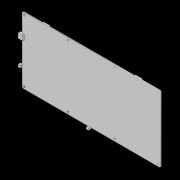
# Autodesk Inventor part: seaboard-block-circuit-board
Saved by Autodesk Inventor 2020 (Build 240168000, 168)
## iProperties
Created: 2019-06-07
Part Number: seaboard-block-circuit-board
Material: Generic
Document SubType Name: Modeling
Designer: valer
Density: 1 g/cm^3
Appearance: Default
Author: valer
Autodesk Inventor part; units mm, degrees
ref_plane "YZ Plane" through (0, 0, 0) normal (1, 0, 0) x (0, 1, 0)
ref_plane "XZ Plane" through (0, 0, 0) normal (0, 1, 0) x (-1, 0, 0)
ref_plane "XY Plane" through (0, 0, 0) normal (0, 0, 1) x (1, 0, 0)
sketch "CircuitBoard" plane through (0, 0, 0) normal (0, 0, 1) x (1, 0, 0)
  line L0 (-271.4625, 131.7625) -> (-267.0175, 131.7625) construction
  line L1 (0, 129.3813) -> (0, 5.9531)
  line L2 (0, 0) -> (-267.0175, 0) construction
  line L3 (-271.4625, 0) -> (-271.4625, 131.7625) construction
  line L4 (-271.4625, 95.25) -> (-267.0175, 95.25)
  line L5 (-267.0175, 95.25) -> (-267.0175, 86.1219) construction
  line L6 (-267.0175, 86.1219) -> (-271.4625, 86.1219)
  line L7 (-271.4625, 86.1219) -> (-271.4625, 95.25)
  line L8 (-271.4625, 95.25) -> (-262.3344, 95.25)
  line L9 (-262.3344, 95.25) -> (-262.3344, 86.1219)
  line L10 (-262.3344, 86.1219) -> (-271.4625, 86.1219)
  line L11 (-271.4625, 86.1219) -> (-271.4625, 95.25)
  line L12 (-267.0175, 95.25) -> (-267.0175, 129.3813)
  line L13 (-264.6363, 131.7625) -> (-2.3812, 131.7625)
  line L14 (-267.0175, 86.1219) -> (-267.0175, 5.9531)
  line L15 (-267.0175, 0) -> (-271.4625, 0) construction
  line L16 (-135.255, 0) -> (-140.0175, 0)
  line L17 (-140.0175, 0) -> (-140.0175, 3.5719)
  line L18 (-140.0175, 3.5719) -> (-135.255, 3.5719)
  line L19 (-135.255, 3.5719) -> (-135.255, 0)
  line L20 (-140.0175, 0) -> (-135.255, 0)
  line L21 (-135.255, 0) -> (-135.255, -1.5875)
  line L22 (-135.255, -1.5875) -> (-140.0175, -1.5875)
  line L23 (-140.0175, -1.5875) -> (-140.0175, 0)
  line L24 (-271.4625, 42.8625) -> (-267.0175, 42.8625)
  line L25 (-267.0175, 42.8625) -> (-267.0175, 38.1)
  line L26 (-267.0175, 38.1) -> (-271.4625, 38.1)
  line L27 (-271.4625, 38.1) -> (-271.4625, 42.8625)
  circle A0 centre (-262.8456, 127.5906) radius 1.7859
  arc A1 (-264.6363, 131.7625) -> (-267.0175, 129.3813) centre (-264.6362, 129.3813) ccw
  arc A2 (0, 129.3813) -> (-2.3812, 131.7625) centre (-2.3812, 129.3813) ccw
  circle A3 centre (-178.7081, 127.5906) radius 1.7859
  line L28 (-262.8456, 127.5906) -> (-178.7081, 127.5906) construction
  line L29 (-271.4625, 42.8625) -> (-273.05, 42.8625)
  line L30 (-273.05, 42.8625) -> (-273.05, 38.1)
  line L31 (-273.05, 38.1) -> (-271.4625, 38.1)
  line L32 (-271.4625, 38.1) -> (-271.4625, 42.8625)
  line L33 (-140.0175, 3.5719) -> (-264.6363, 3.5719)
  line L34 (-135.255, 3.5719) -> (-2.3813, 3.5719)
  line L35 (0, 3.5719) -> (0, 0) construction
  arc A4 (-267.0175, 5.9531) -> (-264.6363, 3.5719) centre (-264.6362, 5.9531) ccw
  arc A5 (-2.3813, 3.5719) -> (0, 5.9531) centre (-2.3813, 5.9531) ccw
  line L36 (-267.0175, 67.6672) -> (0, 67.6672) construction
  line L37 (-133.5087, 131.7625) -> (-133.5088, 3.5719) construction
  circle A6 centre (-4.1719, 127.5906) radius 1.7859
  circle A7 centre (-88.3094, 127.5906) radius 1.7859
  circle A8 centre (-262.8456, 7.7438) radius 1.7859
  circle A9 centre (-178.708, 7.7438) radius 1.7859
  circle A10 centre (-4.1719, 7.7438) radius 1.7859
  circle A11 centre (-88.3094, 7.7438) radius 1.7859
  point P0 (0, 131.7625)
  point P1 (-133.5088, 67.6672)
  dimension "d44" = 271.4625
  dimension "d45" = 131.7625
  dimension "d46" = 4.445
  dimension "d47" = 9.1281
  dimension "d48" = 36.5125
  dimension "d49" = 9.1281
  dimension "d50" = 131.7625
  dimension "d51" = 4.7625
  dimension "d52" = 3.5719
  dimension "d53" = 1.5875
  dimension "d54" = 4.7625
  dimension "d55" = 38.1
  dimension "d56" = 3.5719
  dimension "d57" = 4.1719
  dimension "d58" = 4.1719
  dimension "d59" = 2.3813
  dimension "d60" = 84.1375
  dimension "d61" = 1.5875
  dimension "d62" = 2.3813
  dimension "d65" = 88.3094
  constraints: 77 end point, 20 parallel, 14 point on line, 12 centre point, 9 horizontal, 9 perpendicular, 8 point on circle, 8 tangent, 6 symmetric about line, 4 midpoint, 3 collinear, 3 equal radius, 3 vertical, 1 coincident, 6 other
  measures "d44" distance of L0.start point (0, 131.763)
  measures "d45" distance of L3.start L0.start
  measures "d46" distance of L4.start L4.end
  measures "d47" distance of L4.start L8.end
  measures "d48" distance between parallel lines of L8 L0
  measures "d49" distance of L8.end L9.end
  measures "d50" distance between parallel lines of L14 L19
  measures "d51" distance of L17.end L18.end
  measures "d52" distance of L18.end L16.start
  measures "d53" distance of L22.end L16.end
  measures "d54" distance between parallel lines of L26 L24
  measures "d55" distance between parallel lines of L26 L2
  measures "d56" diameter of A0
  measures "d57" distance from line of L13 L28.start
  measures "d58" distance from line of L12 L28.start
  measures "d59" radius of A1
  measures "d60" distance of L28.start L28.end
  measures "d61" distance of L24.start L29.end
  measures "d62" radius of A4
  measures "d65" distance from line of L1 A11.centre
extrude "CircuitBoardFeature" add sketch "CircuitBoard" along normal blind 1.5875 contours L1 A5 L34 L18 L33 A4 L14 L10 L9 L8 L12 A1 L13 A2 | L19 L16 L17 L18 | L8 L9 L10 L6 L7 L4 | L26 L27 L24 L14
extrude "TopFeatures" add sketch "CircuitBoard" along normal blind 5.08 contours L19 L16 L17 L18 | L8 L9 L10 L6 L7 L4 | L26 L27 L24 L14
sketch "BottomProfile" plane through (0, 0, 0) normal (0, 0, -1) x (-1, 0, 0)
  line L0 (264.6363, 3.5719) -> (140.0175, 3.5719) construction
  line L1 (228.9175, 3.5719) -> (216.2175, 3.5719)
  line L2 (216.2175, 3.5719) -> (216.2175, 11.1919)
  line L3 (216.2175, 11.1919) -> (228.9175, 11.1919)
  line L4 (228.9175, 11.1919) -> (228.9175, 3.5719)
  line L5 (135.255, 3.5719) -> (2.3813, 3.5719) construction
  line L6 (50.8, 3.5719) -> (38.1, 3.5719)
  line L7 (38.1, 3.5719) -> (38.1, 11.1919)
  line L8 (38.1, 11.1919) -> (50.8, 11.1919)
  line L9 (50.8, 11.1919) -> (50.8, 3.5719)
  line L10 (0, 5.9531) -> (0, 129.3813) construction
  line L11 (0, 67.6672) -> (267.0175, 67.6672) construction
  line L12 (267.0175, 86.1219) -> (267.0175, 42.8625) projected
  line L13 (267.0175, 38.1) -> (267.0175, 5.9531) projected
  line L14 (228.9175, 131.7625) -> (216.2175, 131.7625)
  line L15 (216.2175, 131.7625) -> (216.2175, 124.1425)
  line L16 (216.2175, 124.1425) -> (228.9175, 124.1425)
  line L17 (228.9175, 124.1425) -> (228.9175, 131.7625)
  line L18 (50.8, 131.7625) -> (38.1, 131.7625)
  line L19 (38.1, 131.7625) -> (38.1, 124.1425)
  line L20 (38.1, 124.1425) -> (50.8, 124.1425)
  line L21 (50.8, 124.1425) -> (50.8, 131.7625)
  point P0 (0, 0)
  dimension "d70" = 38.1
  dimension "d71" = 38.1
  dimension "d72" = 12.7
  dimension "d73" = 7.62
  constraints: 34 end point, 8 symmetric about line, 5 point on line, 4 parallel, 3 perpendicular, 2 horizontal, 1 collinear, 1 midpoint
  measures "d70" distance between parallel lines of L4 L13
  measures "d71" distance between parallel lines of L10 L7
  measures "d72" distance of L2.end L3.end
  measures "d73" distance of L3.end L1.start
extrude "BottomFeatures" add sketch "BottomProfile" along normal blind 1.5875
equation "\"d58\" = d57"
body "Solid1"
